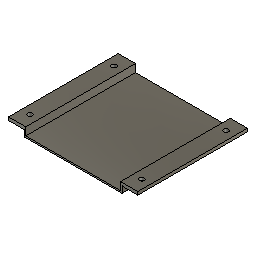
1-CBA bottom Cover V3 - part 3of3 v1 (Autodesk Fusion 360 design; units mm, degrees)
Autodesk Fusion 360 part; units mm, degrees
sketch "extrusion" plane through (0, 0, 0) normal (0, 1, 0) x (1, 0, 0)
  line L0 (-82.5, -8) -> (-62.5, -8)
  line L1 (-62.5, -8) -> (-62.5, 0)
  line L2 (-62.5, 0) -> (62.5, 0)
  line L3 (62.5, 0) -> (62.5, -8)
  line L4 (62.5, -8) -> (82.5, -8)
  line L5 (-60.5, -12) -> (-60.5, -2)
  line L6 (-60.5, -2) -> (60.5, -2)
  line L7 (60.5, -2) -> (60.5, -12)
  line L8 (-82.5, -12) -> (-60.5, -12)
  line L9 (60.5, -12) -> (82.5, -12)
  line L10 (-82.5, -8) -> (-82.5, -12)
  line L11 (82.5, -8) -> (82.5, -12)
  dimension "d1" = 125
  dimension "d2" = 8
  dimension "d3" = 20
  dimension "d4" = 8
  dimension "d5" = 20
  measures "d2" distance of origin
  measures "d4" distance of origin
extrude "Extrude1" add sketch "extrusion" along normal mid plane 140
sketch "top holes" plane through (0, 0, 12) normal (0, 0, 1) x (-1, 0, 0)
  circle A0 centre (71.5, -53.75) radius 3
  line L0 (82.5, -70) -> (60.5, -70)
  dimension "d11" = 6
  dimension "d12" = 16.25
  measures "d11" diameter of A0
extrude "Extrude2" cut sketch "top holes" against normal blind 4
mirror "Mirror1" about plane through (0, 0, 0) normal (1, 0, 0) of "Extrude2"
mirror "Mirror2" about plane through (0, 0, 0) normal (0, 1, 0) of "Extrude2", "Mirror1"
